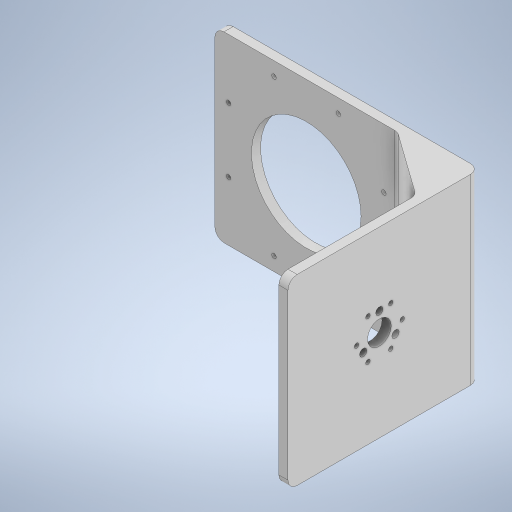
# Autodesk Inventor part: l_r_wp2wr__legparts_07(four)
Saved by Autodesk Inventor 2024.3 (Build 283343000, 343)
## iProperties
Created: 2024-10-21
Part Number: l_r_wp2wr__legparts_07(four)
Material: 一般
Document SubType Name: Modeling
Designer: 佐藤智貴
Density: 1 g/cm^3
Appearance: 既定
Mass: 398.337 g
Surface Area: 461.43 cm^2
Volume: 147.532 cm^3
Author: 佐藤智貴
Autodesk Inventor part; units mm, degrees
ref_plane "YZ Plane" through (0, 0, 0) normal (1, 0, 0) x (0, 1, 0)
ref_plane "XZ Plane" through (0, 0, 0) normal (0, 1, 0) x (-1, 0, 0)
ref_plane "XY Plane" through (0, 0, 0) normal (0, 0, 1) x (1, 0, 0)
sketch "スケッチ1" plane through (0, 0, 0) normal (0, 0, 1) x (1, 0, 0)
  circle A0 centre (0, 0) radius 48.5
  circle A1 centre (0, 0) radius 46.0893
  line L0 (-50, 50) -> (50, 50)
  line L1 (50, 50) -> (50, -50)
  line L2 (50, -50) -> (-50, -50)
  line L3 (-50, -50) -> (-50, 50)
  dimension "d0" = 97
  dimension "d3" = 50
  dimension "d4" = 50
  dimension "d5" = 50
  dimension "d6" = 50
  constraints: 8 end point, 2 centre point, 2 parallel, 1 coincident, 1 horizontal, 1 perpendicular
  measures "d0" diameter of A0
  measures "d3" distance from line of L0 point (0, 0)
  measures "d4" distance from line of L2 point (0, 0)
  measures "d5" distance from line of L1 point (0, 0)
  measures "d6" distance from line of point (0, 0) L3
extrude "押し出し1" add sketch "スケッチ1" along normal blind 5 contours A0 | A1 | L0 L1 L2 L3
sketch "スケッチ2" plane through (0, 0, 5) normal (0, 0, 1) x (1, 0, 0)
  circle A0 centre (0, 0) radius 46
  line L0 (0, 0) -> (0, 64.6511)
  line L1 (0, 0) -> (-25.9524, 62.6547)
  line L2 (-50, 50) -> (-50, -50) projected
  point P0 (-17.6034, 42.4985)
  point P1 (-42.4985, 17.6034)
  point P2 (-42.4985, -17.6034)
  point P3 (-17.6034, -42.4985)
  point P4 (17.6034, -42.4985)
  point P5 (42.4985, -17.6034)
  point P6 (42.4985, 17.6034)
  point P7 (17.6034, 42.4985)
  dimension "d7" = 92
  dimension "d8" = 22.5
  dimension "d11" = 360
  dimension "d76" = 50
  constraints: 4 end point, 1 coincident, 1 point on line, 1 vertical, 12 other
  measures "d8" angle of L0 L1
  measures "d76" distance from line of L2 point (0, 0)
hole "穴1" at (-17.6034, 42.4985, 5) at (-42.4985, 17.6034, 5) at (-42.4985, -17.6034, 5) at (-17.6034, -42.4985, 5) at (17.6034, -42.4985, 5) at (42.4985, -17.6034, 5) at (42.4985, 17.6034, 5) at (17.6034, 42.4985, 5) direction (0, 0, -1) diameter 2.459 end through all
sketch "スケッチ3" plane through (0, 0, 5) normal (0, 0, 1) x (1, 0, 0)
  circle A0 centre (0, 0) radius 30
  dimension "d20" = 60
  constraints: 1 centre point, 1 coincident
  measures "d20" diameter of A0
extrude "押し出し2" cut sketch "スケッチ3" against normal blind 5
sketch "スケッチ4" plane through (50, -50, 0) normal (1, 0, 0) x (0, 0, -1)
  line L0 (-5, 100) -> (-5, 0) projected
  line L1 (-5, 100) -> (0, 100)
  line L2 (0, 100) -> (0, 0)
  line L3 (0, 0) -> (-5, 0)
  line L4 (-5, 0) -> (-5, 100)
  point P0 (0, 50)
  constraints: 8 end point, 2 parallel, 1 horizontal, 1 perpendicular
extrude "押し出し3" add sketch "スケッチ4" along normal blind 40
sketch "スケッチ5" plane through (0, 0, 5) normal (0, 0, 1) x (1, 0, 0)
  line L0 (-50, 50) -> (90, 50) projected
  line L1 (85, 50) -> (90, 50)
  line L2 (90, 50) -> (90, -50)
  line L3 (90, -50) -> (85, -50)
  line L4 (85, -50) -> (85, 50)
  line L5 (-50, -50) -> (90, -50) projected
  line L6 (90, 50) -> (90, -50) projected
  point P0 (0, 0)
  point P1 (90, 50)
  point P2 (90, 0)
  dimension "d25" = 0
  dimension "d26" = 5
  dimension "d27" = 100
  dimension "d70" = 0
  constraints: 8 end point, 2 parallel, 1 horizontal, 1 midpoint, 1 perpendicular, 1 point on line
  measures "d25" distance from line of L5 L2.end
  measures "d26" distance between parallel lines of L2 L4
  measures "d27" distance of L1.end L2.end
  measures "d70" distance from line of L6 point (90, 0)
extrude "押し出し4" add sketch "スケッチ5" along normal blind 100
sketch "スケッチ6" plane through (90, -50, 0) normal (1, 0, 0) x (0, 0, -1)
  circle A0 centre (-55, 50) radius 46
  line L0 (0, 0) -> (-105, 0) projected
  line L1 (0, 0) -> (0, 100) projected
  line L2 (-55, 50) -> (41.9537, 50)
  line L3 (-55, 50) -> (-55, 131.7305)
  line L4 (-55, 50) -> (-80.0101, 110.3797)
  circle A1 centre (-55, 50) radius 12.5
  line L5 (-55, 50) -> (-63.1841, 64.1753)
  point P0 (0, 50)
  point P1 (-72.6034, 92.4985)
  point P2 (-97.4985, 67.6034)
  point P3 (-97.4985, 32.3966)
  point P4 (-72.6034, 7.5015)
  point P5 (-37.3966, 7.5015)
  point P6 (-12.5015, 32.3966)
  point P7 (-12.5015, 67.6034)
  point P8 (-37.3966, 92.4985)
  point P9 (-61.25, 60.8253)
  point P10 (-67.5, 50)
  point P11 (-61.25, 39.1747)
  point P12 (-48.75, 39.1747)
  point P13 (-42.5, 50)
  point P14 (-48.75, 60.8253)
  dimension "d32" = 92
  dimension "d34" = 25
  dimension "d30" = 50
  dimension "d31" = 55
  dimension "d33" = 22.5
  dimension "d35" = 30
  dimension "d38" = 360
  dimension "d42" = 360
  constraints: 8 end point, 2 point on line, 1 coincident, 1 horizontal, 1 vertical, 22 other
  measures "d30" distance from line of L0 L2.start
  measures "d31" distance from line of L1 L2.start
  measures "d33" angle of L4 L3
  measures "d35" angle of L3 L5
hole "穴2" at (90, 10.8253, 48.75) at (90, 10.8253, 61.25) at (90, 0, 67.5) at (90, 0, 42.5) at (90, -10.8253, 48.75) at (90, -10.8253, 61.25) direction (-1, 0, 0) diameter 2.459 end through all
sketch "スケッチ7" plane through (90, -50, 0) normal (1, 0, 0) x (0, 0, -1)
  line L0 (-55, 50) -> (26.223, 50)
  circle A0 centre (-55, 50) radius 10.2
  line L1 (0, 0) -> (0, 100) projected
  line L2 (0, 0) -> (-105, 0) projected
  line L3 (-55, 50) -> (-55, 82.0983)
  point P0 (0, 50)
  point P1 (-55, 60.2)
  point P2 (-63.8335, 44.9)
  point P3 (-46.1665, 44.9)
  dimension "d53" = 20.4
  dimension "d51" = 55
  dimension "d52" = 50
  dimension "d56" = 360
  constraints: 4 end point, 1 coincident, 1 horizontal, 1 point on line, 1 vertical, 1 vertical alignment, 6 other
  measures "d51" distance from line of L1 L3.start
  measures "d52" distance from line of L2 L3.start
hole "穴3" at (90, 10.2, 55) at (90, -5.1, 63.8335) at (90, -5.1, 46.1665) direction (-1, 0, 0) diameter 4 end through all
sketch "スケッチ8" plane through (90, -50, 0) normal (1, 0, 0) x (0, 0, -1)
  circle A0 centre (-55, 50) radius 6.5
  line L0 (0, 0) -> (0, 100) projected
  line L1 (0, 0) -> (-105, 0) projected
  point P0 (0, 50)
  dimension "d65" = 13
  dimension "d66" = 55
  dimension "d67" = 50
  constraints: 1 centre point
  measures "d65" diameter of A0
  measures "d66" distance from line of L0 A0.centre
  measures "d67" distance from line of L1 A0.centre
extrude "押し出し5" cut sketch "スケッチ8" against normal through all
sketch "スケッチ13" plane through (0, 0, 0) normal (0, 1, 0) x (-1, 0, 0)
  line L0 (-90, 0) -> (-50, 0)
  line L1 (-50, 0) -> (-50, 30)
  line L2 (-50, 30) -> (-90, 30)
  line L3 (-90, 30) -> (-90, 0)
  line L4 (-90, 0) -> (-90, 105) projected
  line L5 (50, 0) -> (-90, 0) projected
  arc A0 (-85, 10) -> (-80, 5) centre (-80, 10) ccw projected
  line L6 (-80, 5) -> (-46.2653, 5)
  line L7 (-50, 5) -> (-85, 30)
  point P0 (0, 0)
  point P1 (-90, 5)
  point P2 (-90, 100)
  point P3 (45, 0)
  point P4 (-85, 0)
  dimension "d92" = 40
  dimension "d93" = 0
  dimension "d94" = 30
  dimension "d95" = 0
  constraints: 12 end point, 3 point on line, 2 horizontal, 2 parallel, 1 perpendicular, 1 tangent
  measures "d92" distance from line of L3 L1.end
  measures "d93" distance between parallel lines of L4 L3
  measures "d94" distance between parallel lines of L2 L0
  measures "d95" distance between parallel lines of L0 L5
extrude "押し出し9" add sketch "スケッチ13" along normal mid plane 100 contours L3 L2 L7 L1 L0
fillet "フィレット2" radius 5 7 edges at (-50, -50, 2.5) (-50, 50, 2.5) (85, 0, 30) (90, 0, 0) (50, 0, 5) (87.5, -50, 105) (87.5, 50, 105)
sketch "スケッチ16" plane through (0, 0, 0) normal (0, 0, -1) x (-1, 0, 0)
  circle A0 centre (17.6034, 42.4985) radius 1.2295 projected
  circle A1 centre (0, 0) radius 46
  circle A2 centre (17.6034, 42.4985) radius 3
  circle A3 centre (-17.6034, 42.4985) radius 3
  circle A4 centre (-42.4985, 17.6034) radius 3
  circle A5 centre (-42.4985, -17.6034) radius 3
  circle A6 centre (-17.6034, -42.4985) radius 3
  circle A7 centre (17.6034, -42.4985) radius 3
  circle A8 centre (42.4985, -17.6034) radius 3
  circle A9 centre (42.4985, 17.6034) radius 3
  dimension "d113" = 6
  dimension "d116" = 360
  constraints: 8 centre point, 2 coincident, 20 other
  measures "d113" diameter of A2
extrude "押し出し12" cut sketch "スケッチ16" against normal blind 2 contours A0 A1 | A0 A1 A2 | A1 A0 | A0 A1 A2 | A3 A1 | A1 A3 | A9 A1 | A1 A9 | A4 A1 | A1 A4 | A8 A1 | A1 A8 | A5 A1 | A1 A5 | A7 A1 | A1 A7 | A6 A1 | A1 A6
equation "\"d4\" = d3"
equation "\"d5\" = d3"
equation "\"d6\" = d5"
